Autodesk Inventor part; units mm, degrees
(part 4 of 6)
  line L241 (-272.47, 0.63) -> (-272.9893, 0.63)
  arc A1710 (-273.138, 0.7604) -> (-272.9893, 0.63) centre (-272.9893, 0.78) ccw
  arc A1711 (-273.138, 0.7604) -> (-273.2306, 1.0682) centre (-274.1294, 0.63) ccw
  arc A1712 (-273.2306, 1.0682) -> (-273.7296, 1.38) centre (-273.7294, 0.825) ccw
  arc A1713 (-273.7296, 1.38) -> (-274.2287, 1.0682) centre (-273.7298, 0.825) ccw
  arc A1714 (-274.2287, 1.0682) -> (-274.3213, 0.7604) centre (-273.3298, 0.63) ccw
  arc A1715 (-274.47, 0.63) -> (-274.3213, 0.7604) centre (-274.47, 0.78) ccw
  line L242 (-274.47, 0.63) -> (-274.9893, 0.63)
  arc A1716 (-275.138, 0.7604) -> (-274.9893, 0.63) centre (-274.9893, 0.78) ccw
  arc A1717 (-275.138, 0.7604) -> (-275.2306, 1.0682) centre (-276.1294, 0.63) ccw
  arc A1718 (-275.2306, 1.0682) -> (-275.7296, 1.38) centre (-275.7294, 0.825) ccw
  arc A1719 (-275.7296, 1.38) -> (-276.2287, 1.0682) centre (-275.7298, 0.825) ccw
  arc A1720 (-276.2287, 1.0682) -> (-276.3213, 0.7604) centre (-275.3298, 0.63) ccw
  arc A1721 (-276.47, 0.63) -> (-276.3213, 0.7604) centre (-276.47, 0.78) ccw
  line L243 (-276.47, 0.63) -> (-276.9893, 0.63)
  arc A1722 (-277.138, 0.7604) -> (-276.9893, 0.63) centre (-276.9893, 0.78) ccw
  arc A1723 (-277.138, 0.7604) -> (-277.2306, 1.0682) centre (-278.1294, 0.63) ccw
  arc A1724 (-277.2306, 1.0682) -> (-277.7296, 1.38) centre (-277.7294, 0.825) ccw
  arc A1725 (-277.7296, 1.38) -> (-278.2287, 1.0682) centre (-277.7298, 0.825) ccw
  arc A1726 (-278.2287, 1.0682) -> (-278.3213, 0.7604) centre (-277.3298, 0.63) ccw
  arc A1727 (-278.47, 0.63) -> (-278.3213, 0.7604) centre (-278.47, 0.78) ccw
  line L244 (-278.47, 0.63) -> (-278.9893, 0.63)
  arc A1728 (-279.138, 0.7604) -> (-278.9893, 0.63) centre (-278.9893, 0.78) ccw
  arc A1729 (-279.138, 0.7604) -> (-279.2306, 1.0682) centre (-280.1294, 0.63) ccw
  arc A1730 (-279.2306, 1.0682) -> (-279.7296, 1.38) centre (-279.7294, 0.825) ccw
  arc A1731 (-279.7296, 1.38) -> (-280.2287, 1.0682) centre (-279.7298, 0.825) ccw
  arc A1732 (-280.2287, 1.0682) -> (-280.3213, 0.7604) centre (-279.3298, 0.63) ccw
  arc A1733 (-280.47, 0.63) -> (-280.3213, 0.7604) centre (-280.47, 0.78) ccw
  line L245 (-280.47, 0.63) -> (-280.9893, 0.63)
  arc A1734 (-281.138, 0.7604) -> (-280.9893, 0.63) centre (-280.9893, 0.78) ccw
  arc A1735 (-281.138, 0.7604) -> (-281.2306, 1.0682) centre (-282.1294, 0.63) ccw
  arc A1736 (-281.2306, 1.0682) -> (-281.7296, 1.38) centre (-281.7294, 0.825) ccw
  arc A1737 (-281.7296, 1.38) -> (-282.2287, 1.0682) centre (-281.7298, 0.825) ccw
  arc A1738 (-282.2287, 1.0682) -> (-282.3213, 0.7604) centre (-281.3298, 0.63) ccw
  arc A1739 (-282.47, 0.63) -> (-282.3213, 0.7604) centre (-282.47, 0.78) ccw
  line L246 (-282.47, 0.63) -> (-282.9893, 0.63)
  arc A1740 (-283.138, 0.7604) -> (-282.9893, 0.63) centre (-282.9893, 0.78) ccw
  arc A1741 (-283.138, 0.7604) -> (-283.2306, 1.0682) centre (-284.1294, 0.63) ccw
  arc A1742 (-283.2306, 1.0682) -> (-283.7296, 1.38) centre (-283.7294, 0.825) ccw
  arc A1743 (-283.7296, 1.38) -> (-284.2287, 1.0682) centre (-283.7298, 0.825) ccw
  arc A1744 (-284.2287, 1.0682) -> (-284.3213, 0.7604) centre (-283.3298, 0.63) ccw
  arc A1745 (-284.47, 0.63) -> (-284.3213, 0.7604) centre (-284.47, 0.78) ccw
  line L247 (-284.47, 0.63) -> (-284.9893, 0.63)
  arc A1746 (-285.138, 0.7604) -> (-284.9893, 0.63) centre (-284.9893, 0.78) ccw
  arc A1747 (-285.138, 0.7604) -> (-285.2306, 1.0682) centre (-286.1294, 0.63) ccw
  arc A1748 (-285.2306, 1.0682) -> (-285.7296, 1.38) centre (-285.7294, 0.825) ccw
  arc A1749 (-285.7296, 1.38) -> (-286.2287, 1.0682) centre (-285.7298, 0.825) ccw
  arc A1750 (-286.2287, 1.0682) -> (-286.3213, 0.7604) centre (-285.3298, 0.63) ccw
  arc A1751 (-286.47, 0.63) -> (-286.3213, 0.7604) centre (-286.47, 0.78) ccw
  line L248 (-286.47, 0.63) -> (-286.9893, 0.63)
  arc A1752 (-287.138, 0.7604) -> (-286.9893, 0.63) centre (-286.9893, 0.78) ccw
  arc A1753 (-287.138, 0.7604) -> (-287.2306, 1.0682) centre (-288.1294, 0.63) ccw
  arc A1754 (-287.2306, 1.0682) -> (-287.7296, 1.38) centre (-287.7294, 0.825) ccw
  arc A1755 (-287.7296, 1.38) -> (-288.2287, 1.0682) centre (-287.7298, 0.825) ccw
  arc A1756 (-288.2287, 1.0682) -> (-288.3213, 0.7604) centre (-287.3298, 0.63) ccw
  arc A1757 (-288.47, 0.63) -> (-288.3213, 0.7604) centre (-288.47, 0.78) ccw
  line L249 (-288.47, 0.63) -> (-288.9893, 0.63)
  arc A1758 (-289.138, 0.7604) -> (-288.9893, 0.63) centre (-288.9893, 0.78) ccw
  arc A1759 (-289.138, 0.7604) -> (-289.2306, 1.0682) centre (-290.1294, 0.63) ccw
  arc A1760 (-289.2306, 1.0682) -> (-289.7296, 1.38) centre (-289.7294, 0.825) ccw
  arc A1761 (-289.7296, 1.38) -> (-290.2287, 1.0682) centre (-289.7298, 0.825) ccw
  arc A1762 (-290.2287, 1.0682) -> (-290.3213, 0.7604) centre (-289.3298, 0.63) ccw
  arc A1763 (-290.47, 0.63) -> (-290.3213, 0.7604) centre (-290.47, 0.78) ccw
  line L250 (-290.47, 0.63) -> (-290.9893, 0.63)
  arc A1764 (-291.138, 0.7604) -> (-290.9893, 0.63) centre (-290.9893, 0.78) ccw
  arc A1765 (-291.138, 0.7604) -> (-291.2306, 1.0682) centre (-292.1294, 0.63) ccw
  arc A1766 (-291.2306, 1.0682) -> (-291.7296, 1.38) centre (-291.7294, 0.825) ccw
  arc A1767 (-291.7296, 1.38) -> (-292.2287, 1.0682) centre (-291.7298, 0.825) ccw
  arc A1768 (-292.2287, 1.0682) -> (-292.3213, 0.7604) centre (-291.3298, 0.63) ccw
  arc A1769 (-292.47, 0.63) -> (-292.3213, 0.7604) centre (-292.47, 0.78) ccw
  line L251 (-292.47, 0.63) -> (-292.9893, 0.63)
  arc A1770 (-293.138, 0.7604) -> (-292.9893, 0.63) centre (-292.9893, 0.78) ccw
  arc A1771 (-293.138, 0.7604) -> (-293.2306, 1.0682) centre (-294.1294, 0.63) ccw
  arc A1772 (-293.2306, 1.0682) -> (-293.7296, 1.38) centre (-293.7294, 0.825) ccw
  arc A1773 (-293.7296, 1.38) -> (-294.2287, 1.0682) centre (-293.7298, 0.825) ccw
  arc A1774 (-294.2287, 1.0682) -> (-294.3213, 0.7604) centre (-293.3298, 0.63) ccw
  arc A1775 (-294.47, 0.63) -> (-294.3213, 0.7604) centre (-294.47, 0.78) ccw
  line L252 (-294.47, 0.63) -> (-294.9893, 0.63)
  arc A1776 (-295.138, 0.7604) -> (-294.9893, 0.63) centre (-294.9893, 0.78) ccw
  arc A1777 (-295.138, 0.7604) -> (-295.2306, 1.0682) centre (-296.1294, 0.63) ccw
  arc A1778 (-295.2306, 1.0682) -> (-295.7296, 1.38) centre (-295.7294, 0.825) ccw
  arc A1779 (-295.7296, 1.38) -> (-296.2287, 1.0682) centre (-295.7298, 0.825) ccw
  arc A1780 (-296.2287, 1.0682) -> (-296.3213, 0.7604) centre (-295.3298, 0.63) ccw
  arc A1781 (-296.47, 0.63) -> (-296.3213, 0.7604) centre (-296.47, 0.78) ccw
  line L253 (-296.47, 0.63) -> (-296.9893, 0.63)
  arc A1782 (-297.138, 0.7604) -> (-296.9893, 0.63) centre (-296.9893, 0.78) ccw
  arc A1783 (-297.138, 0.7604) -> (-297.2306, 1.0682) centre (-298.1294, 0.63) ccw
  arc A1784 (-297.2306, 1.0682) -> (-297.7296, 1.38) centre (-297.7294, 0.825) ccw
  arc A1785 (-297.7296, 1.38) -> (-298.2287, 1.0682) centre (-297.7298, 0.825) ccw
  arc A1786 (-298.2287, 1.0682) -> (-298.3213, 0.7604) centre (-297.3298, 0.63) ccw
  arc A1787 (-298.47, 0.63) -> (-298.3213, 0.7604) centre (-298.47, 0.78) ccw
  line L254 (-298.47, 0.63) -> (-298.9893, 0.63)
  arc A1788 (-299.138, 0.7604) -> (-298.9893, 0.63) centre (-298.9893, 0.78) ccw
  arc A1789 (-299.138, 0.7604) -> (-299.2306, 1.0682) centre (-300.1294, 0.63) ccw
  arc A1790 (-299.2306, 1.0682) -> (-299.7296, 1.38) centre (-299.7294, 0.825) ccw
  arc A1791 (-299.7296, 1.38) -> (-300.2287, 1.0682) centre (-299.7298, 0.825) ccw
  arc A1792 (-300.2287, 1.0682) -> (-300.3213, 0.7604) centre (-299.3298, 0.63) ccw
  arc A1793 (-300.47, 0.63) -> (-300.3213, 0.7604) centre (-300.47, 0.78) ccw
  line L255 (-300.47, 0.63) -> (-300.9893, 0.63)
  arc A1794 (-301.138, 0.7604) -> (-300.9893, 0.63) centre (-300.9893, 0.78) ccw
  arc A1795 (-301.138, 0.7604) -> (-301.2306, 1.0682) centre (-302.1294, 0.63) ccw
  arc A1796 (-301.2306, 1.0682) -> (-301.7296, 1.38) centre (-301.7294, 0.825) ccw
  arc A1797 (-301.7296, 1.38) -> (-302.2287, 1.0682) centre (-301.7298, 0.825) ccw
  arc A1798 (-302.2287, 1.0682) -> (-302.3213, 0.7604) centre (-301.3298, 0.63) ccw
  arc A1799 (-302.47, 0.63) -> (-302.3213, 0.7604) centre (-302.47, 0.78) ccw
  line L256 (-302.47, 0.63) -> (-302.9893, 0.63)
  arc A1800 (-303.138, 0.7604) -> (-302.9893, 0.63) centre (-302.9893, 0.78) ccw
  arc A1801 (-303.138, 0.7604) -> (-303.2306, 1.0682) centre (-304.1294, 0.63) ccw
  arc A1802 (-303.2306, 1.0682) -> (-303.7296, 1.38) centre (-303.7294, 0.825) ccw
  arc A1803 (-303.7296, 1.38) -> (-304.2287, 1.0682) centre (-303.7298, 0.825) ccw
  arc A1804 (-304.2287, 1.0682) -> (-304.3213, 0.7604) centre (-303.3298, 0.63) ccw
  arc A1805 (-304.47, 0.63) -> (-304.3213, 0.7604) centre (-304.47, 0.78) ccw
  line L257 (-304.47, 0.63) -> (-304.9893, 0.63)
  arc A1806 (-305.138, 0.7604) -> (-304.9893, 0.63) centre (-304.9893, 0.78) ccw
  arc A1807 (-305.138, 0.7604) -> (-305.2306, 1.0682) centre (-306.1294, 0.63) ccw
  arc A1808 (-305.2306, 1.0682) -> (-305.7296, 1.38) centre (-305.7294, 0.825) ccw
  arc A1809 (-305.7296, 1.38) -> (-306.2287, 1.0682) centre (-305.7298, 0.825) ccw
  arc A1810 (-306.2287, 1.0682) -> (-306.3213, 0.7604) centre (-305.3298, 0.63) ccw
  arc A1811 (-306.47, 0.63) -> (-306.3213, 0.7604) centre (-306.47, 0.78) ccw
  line L258 (-306.47, 0.63) -> (-306.9893, 0.63)
  arc A1812 (-307.138, 0.7604) -> (-306.9893, 0.63) centre (-306.9893, 0.78) ccw
  arc A1813 (-307.138, 0.7604) -> (-307.2306, 1.0682) centre (-308.1294, 0.63) ccw
  arc A1814 (-307.2306, 1.0682) -> (-307.7296, 1.38) centre (-307.7294, 0.825) ccw
  arc A1815 (-307.7296, 1.38) -> (-308.2287, 1.0682) centre (-307.7298, 0.825) ccw
  arc A1816 (-308.2287, 1.0682) -> (-308.3213, 0.7604) centre (-307.3298, 0.63) ccw
  arc A1817 (-308.47, 0.63) -> (-308.3213, 0.7604) centre (-308.47, 0.78) ccw
  line L259 (-308.47, 0.63) -> (-308.9893, 0.63)
  arc A1818 (-309.138, 0.7604) -> (-308.9893, 0.63) centre (-308.9893, 0.78) ccw
  arc A1819 (-309.138, 0.7604) -> (-309.2306, 1.0682) centre (-310.1294, 0.63) ccw
  arc A1820 (-309.2306, 1.0682) -> (-309.7296, 1.38) centre (-309.7294, 0.825) ccw
  arc A1821 (-309.7296, 1.38) -> (-310.2287, 1.0682) centre (-309.7298, 0.825) ccw
  arc A1822 (-310.2287, 1.0682) -> (-310.3213, 0.7604) centre (-309.3298, 0.63) ccw
  arc A1823 (-310.47, 0.63) -> (-310.3213, 0.7604) centre (-310.47, 0.78) ccw
  line L260 (-310.47, 0.63) -> (-310.9893, 0.63)
  arc A1824 (-311.138, 0.7604) -> (-310.9893, 0.63) centre (-310.9893, 0.78) ccw
  arc A1825 (-311.138, 0.7604) -> (-311.2306, 1.0682) centre (-312.1294, 0.63) ccw
  arc A1826 (-311.2306, 1.0682) -> (-311.7296, 1.38) centre (-311.7294, 0.825) ccw
  arc A1827 (-311.7296, 1.38) -> (-312.2287, 1.0682) centre (-311.7298, 0.825) ccw
  arc A1828 (-312.2287, 1.0682) -> (-312.3213, 0.7604) centre (-311.3298, 0.63) ccw
  arc A1829 (-312.47, 0.63) -> (-312.3213, 0.7604) centre (-312.47, 0.78) ccw
  line L261 (-312.47, 0.63) -> (-312.9893, 0.63)
  arc A1830 (-313.138, 0.7604) -> (-312.9893, 0.63) centre (-312.9893, 0.78) ccw
  arc A1831 (-313.138, 0.7604) -> (-313.2306, 1.0682) centre (-314.1294, 0.63) ccw
  arc A1832 (-313.2306, 1.0682) -> (-313.7296, 1.38) centre (-313.7294, 0.825) ccw
  arc A1833 (-313.7296, 1.38) -> (-314.2287, 1.0682) centre (-313.7298, 0.825) ccw
  arc A1834 (-314.2287, 1.0682) -> (-314.3213, 0.7604) centre (-313.3298, 0.63) ccw
  arc A1835 (-314.47, 0.63) -> (-314.3213, 0.7604) centre (-314.47, 0.78) ccw
  line L262 (-314.47, 0.63) -> (-314.9893, 0.63)
  arc A1836 (-315.138, 0.7604) -> (-314.9893, 0.63) centre (-314.9893, 0.78) ccw
  arc A1837 (-315.138, 0.7604) -> (-315.2306, 1.0682) centre (-316.1294, 0.63) ccw
  arc A1838 (-315.2306, 1.0682) -> (-315.7296, 1.38) centre (-315.7294, 0.825) ccw
  arc A1839 (-315.7296, 1.38) -> (-316.2287, 1.0682) centre (-315.7298, 0.825) ccw
  arc A1840 (-316.2287, 1.0682) -> (-316.3213, 0.7604) centre (-315.3298, 0.63) ccw
  arc A1841 (-316.47, 0.63) -> (-316.3213, 0.7604) centre (-316.47, 0.78) ccw
  line L263 (-316.47, 0.63) -> (-316.9893, 0.63)
  arc A1842 (-317.138, 0.7604) -> (-316.9893, 0.63) centre (-316.9893, 0.78) ccw
  arc A1843 (-317.138, 0.7604) -> (-317.2306, 1.0682) centre (-318.1294, 0.63) ccw
  arc A1844 (-317.2306, 1.0682) -> (-317.7296, 1.38) centre (-317.7294, 0.825) ccw
  arc A1845 (-317.7296, 1.38) -> (-318.2287, 1.0682) centre (-317.7298, 0.825) ccw
  arc A1846 (-318.2287, 1.0682) -> (-318.3213, 0.7604) centre (-317.3298, 0.63) ccw
  arc A1847 (-318.47, 0.63) -> (-318.3213, 0.7604) centre (-318.47, 0.78) ccw
  line L264 (-318.47, 0.63) -> (-318.9893, 0.63)
  arc A1848 (-319.138, 0.7604) -> (-318.9893, 0.63) centre (-318.9893, 0.78) ccw
  arc A1849 (-319.138, 0.7604) -> (-319.2306, 1.0682) centre (-320.1294, 0.63) ccw
  arc A1850 (-319.2306, 1.0682) -> (-319.7296, 1.38) centre (-319.7294, 0.825) ccw
  arc A1851 (-319.7296, 1.38) -> (-320.2287, 1.0682) centre (-319.7298, 0.825) ccw
  arc A1852 (-320.2287, 1.0682) -> (-320.3213, 0.7604) centre (-319.3298, 0.63) ccw
  arc A1853 (-320.47, 0.63) -> (-320.3213, 0.7604) centre (-320.47, 0.78) ccw
  line L265 (-320.47, 0.63) -> (-320.9893, 0.63)
  arc A1854 (-321.138, 0.7604) -> (-320.9893, 0.63) centre (-320.9893, 0.78) ccw
  arc A1855 (-321.138, 0.7604) -> (-321.2306, 1.0682) centre (-322.1294, 0.63) ccw
  arc A1856 (-321.2306, 1.0682) -> (-321.7296, 1.38) centre (-321.7294, 0.825) ccw
  arc A1857 (-321.7296, 1.38) -> (-322.2287, 1.0682) centre (-321.7298, 0.825) ccw
  arc A1858 (-322.2287, 1.0682) -> (-322.3213, 0.7604) centre (-321.3298, 0.63) ccw
  arc A1859 (-322.47, 0.63) -> (-322.3213, 0.7604) centre (-322.47, 0.78) ccw
  line L266 (-322.47, 0.63) -> (-322.9893, 0.63)
  arc A1860 (-323.138, 0.7604) -> (-322.9893, 0.63) centre (-322.9893, 0.78) ccw
  arc A1861 (-323.138, 0.7604) -> (-323.2306, 1.0682) centre (-324.1294, 0.63) ccw
  arc A1862 (-323.2306, 1.0682) -> (-323.7296, 1.38) centre (-323.7294, 0.825) ccw
  arc A1863 (-323.7296, 1.38) -> (-324.2287, 1.0682) centre (-323.7298, 0.825) ccw
  arc A1864 (-324.2287, 1.0682) -> (-324.3213, 0.7604) centre (-323.3298, 0.63) ccw
  arc A1865 (-324.47, 0.63) -> (-324.3213, 0.7604) centre (-324.47, 0.78) ccw
  line L267 (-324.47, 0.63) -> (-324.9893, 0.63)
  arc A1866 (-325.138, 0.7604) -> (-324.9893, 0.63) centre (-324.9893, 0.78) ccw
  arc A1867 (-325.138, 0.7604) -> (-325.2306, 1.0682) centre (-326.1294, 0.63) ccw
  arc A1868 (-325.2306, 1.0682) -> (-325.7296, 1.38) centre (-325.7294, 0.825) ccw
  arc A1869 (-325.7296, 1.38) -> (-326.2287, 1.0682) centre (-325.7298, 0.825) ccw
  arc A1870 (-326.2287, 1.0682) -> (-326.3213, 0.7604) centre (-325.3298, 0.63) ccw
  arc A1871 (-326.47, 0.63) -> (-326.3213, 0.7604) centre (-326.47, 0.78) ccw
  line L268 (-326.47, 0.63) -> (-326.9893, 0.63)
  arc A1872 (-327.138, 0.7604) -> (-326.9893, 0.63) centre (-326.9893, 0.78) ccw
  arc A1873 (-327.138, 0.7604) -> (-327.2306, 1.0682) centre (-328.1294, 0.63) ccw
  arc A1874 (-327.2306, 1.0682) -> (-327.7296, 1.38) centre (-327.7294, 0.825) ccw
  arc A1875 (-327.7296, 1.38) -> (-328.2287, 1.0682) centre (-327.7298, 0.825) ccw
  arc A1876 (-328.2287, 1.0682) -> (-328.3213, 0.7604) centre (-327.3298, 0.63) ccw
  arc A1877 (-328.47, 0.63) -> (-328.3213, 0.7604) centre (-328.47, 0.78) ccw
  line L269 (-328.47, 0.63) -> (-328.9893, 0.63)
  arc A1878 (-329.138, 0.7604) -> (-328.9893, 0.63) centre (-328.9893, 0.78) ccw
  arc A1879 (-329.138, 0.7604) -> (-329.2306, 1.0682) centre (-330.1294, 0.63) ccw
  arc A1880 (-329.2306, 1.0682) -> (-329.7296, 1.38) centre (-329.7294, 0.825) ccw
  arc A1881 (-329.7296, 1.38) -> (-330.2287, 1.0682) centre (-329.7298, 0.825) ccw
  arc A1882 (-330.2287, 1.0682) -> (-330.3213, 0.7604) centre (-329.3298, 0.63) ccw
  arc A1883 (-330.47, 0.63) -> (-330.3213, 0.7604) centre (-330.47, 0.78) ccw
  line L270 (-330.47, 0.63) -> (-330.9893, 0.63)
  arc A1884 (-331.138, 0.7604) -> (-330.9893, 0.63) centre (-330.9893, 0.78) ccw
  arc A1885 (-331.138, 0.7604) -> (-331.2306, 1.0682) centre (-332.1294, 0.63) ccw
  arc A1886 (-331.2306, 1.0682) -> (-331.7296, 1.38) centre (-331.7294, 0.825) ccw
  arc A1887 (-331.7296, 1.38) -> (-332.2287, 1.0682) centre (-331.7298, 0.825) ccw
  arc A1888 (-332.2287, 1.0682) -> (-332.3213, 0.7604) centre (-331.3298, 0.63) ccw
  arc A1889 (-332.47, 0.63) -> (-332.3213, 0.7604) centre (-332.47, 0.78) ccw
  line L271 (-332.47, 0.63) -> (-332.9893, 0.63)
  arc A1890 (-333.138, 0.7604) -> (-332.9893, 0.63) centre (-332.9893, 0.78) ccw
  arc A1891 (-333.138, 0.7604) -> (-333.2306, 1.0682) centre (-334.1294, 0.63) ccw
  arc A1892 (-333.2306, 1.0682) -> (-333.7296, 1.38) centre (-333.7294, 0.825) ccw
  arc A1893 (-333.7296, 1.38) -> (-334.2287, 1.0682) centre (-333.7298, 0.825) ccw
  arc A1894 (-334.2287, 1.0682) -> (-334.3213, 0.7604) centre (-333.3298, 0.63) ccw
  arc A1895 (-334.47, 0.63) -> (-334.3213, 0.7604) centre (-334.47, 0.78) ccw
  line L272 (-334.47, 0.63) -> (-334.9893, 0.63)
  arc A1896 (-335.138, 0.7604) -> (-334.9893, 0.63) centre (-334.9893, 0.78) ccw
  arc A1897 (-335.138, 0.7604) -> (-335.2306, 1.0682) centre (-336.1294, 0.63) ccw
  arc A1898 (-335.2306, 1.0682) -> (-335.7296, 1.38) centre (-335.7294, 0.825) ccw
  arc A1899 (-335.7296, 1.38) -> (-336.2287, 1.0682) centre (-335.7298, 0.825) ccw
  arc A1900 (-336.2287, 1.0682) -> (-336.3213, 0.7604) centre (-335.3298, 0.63) ccw
  arc A1901 (-336.47, 0.63) -> (-336.3213, 0.7604) centre (-336.47, 0.78) ccw
  line L273 (-336.47, 0.63) -> (-336.9893, 0.63)
  arc A1902 (-337.138, 0.7604) -> (-336.9893, 0.63) centre (-336.9893, 0.78) ccw
  arc A1903 (-337.138, 0.7604) -> (-337.2306, 1.0682) centre (-338.1294, 0.63) ccw
  arc A1904 (-337.2306, 1.0682) -> (-337.7296, 1.38) centre (-337.7294, 0.825) ccw
  arc A1905 (-337.7296, 1.38) -> (-338.2287, 1.0682) centre (-337.7298, 0.825) ccw
  arc A1906 (-338.2287, 1.0682) -> (-338.3213, 0.7604) centre (-337.3298, 0.63) ccw
  arc A1907 (-338.47, 0.63) -> (-338.3213, 0.7604) centre (-338.47, 0.78) ccw
  line L274 (-338.47, 0.63) -> (-338.9893, 0.63)
  arc A1908 (-339.138, 0.7604) -> (-338.9893, 0.63) centre (-338.9893, 0.78) ccw
  arc A1909 (-339.138, 0.7604) -> (-339.2306, 1.0682) centre (-340.1294, 0.63) ccw
  arc A1910 (-339.2306, 1.0682) -> (-339.7296, 1.38) centre (-339.7294, 0.825) ccw
  arc A1911 (-339.7296, 1.38) -> (-340.2287, 1.0682) centre (-339.7298, 0.825) ccw
  arc A1912 (-340.2287, 1.0682) -> (-340.3213, 0.7604) centre (-339.3298, 0.63) ccw
  arc A1913 (-340.47, 0.63) -> (-340.3213, 0.7604) centre (-340.47, 0.78) ccw
  line L275 (-340.47, 0.63) -> (-340.9893, 0.63)
  arc A1914 (-341.138, 0.7604) -> (-340.9893, 0.63) centre (-340.9893, 0.78) ccw
  arc A1915 (-341.138, 0.7604) -> (-341.2306, 1.0682) centre (-342.1294, 0.63) ccw
  arc A1916 (-341.2306, 1.0682) -> (-341.7296, 1.38) centre (-341.7294, 0.825) ccw
  arc A1917 (-341.7296, 1.38) -> (-342.2287, 1.0682) centre (-341.7298, 0.825) ccw
  arc A1918 (-342.2287, 1.0682) -> (-342.3213, 0.7604) centre (-341.3298, 0.63) ccw
  arc A1919 (-342.47, 0.63) -> (-342.3213, 0.7604) centre (-342.47, 0.78) ccw
  line L276 (-342.47, 0.63) -> (-342.9893, 0.63)
  arc A1920 (-343.138, 0.7604) -> (-342.9893, 0.63) centre (-342.9893, 0.78) ccw
  arc A1921 (-343.138, 0.7604) -> (-343.2306, 1.0682) centre (-344.1294, 0.63) ccw
  arc A1922 (-343.2306, 1.0682) -> (-343.7296, 1.38) centre (-343.7294, 0.825) ccw
  arc A1923 (-343.7296, 1.38) -> (-344.2287, 1.0682) centre (-343.7298, 0.825) ccw
  arc A1924 (-344.2287, 1.0682) -> (-344.3213, 0.7604) centre (-343.3298, 0.63) ccw
  arc A1925 (-344.47, 0.63) -> (-344.3213, 0.7604) centre (-344.47, 0.78) ccw
  line L277 (-344.47, 0.63) -> (-344.9893, 0.63)
  arc A1926 (-345.138, 0.7604) -> (-344.9893, 0.63) centre (-344.9893, 0.78) ccw
  arc A1927 (-345.138, 0.7604) -> (-345.2306, 1.0682) centre (-346.1294, 0.63) ccw
  arc A1928 (-345.2306, 1.0682) -> (-345.7296, 1.38) centre (-345.7294, 0.825) ccw
  arc A1929 (-345.7296, 1.38) -> (-346.2287, 1.0682) centre (-345.7298, 0.825) ccw
  arc A1930 (-346.2287, 1.0682) -> (-346.3213, 0.7604) centre (-345.3298, 0.63) ccw
  arc A1931 (-346.47, 0.63) -> (-346.3213, 0.7604) centre (-346.47, 0.78) ccw
  line L278 (-346.47, 0.63) -> (-346.9893, 0.63)
  arc A1932 (-347.138, 0.7604) -> (-346.9893, 0.63) centre (-346.9893, 0.78) ccw
  arc A1933 (-347.138, 0.7604) -> (-347.2306, 1.0682) centre (-348.1294, 0.63) ccw
  arc A1934 (-347.2306, 1.0682) -> (-347.7296, 1.38) centre (-347.7294, 0.825) ccw
  arc A1935 (-347.7296, 1.38) -> (-348.2287, 1.0682) centre (-347.7298, 0.825) ccw
  arc A1936 (-348.2287, 1.0682) -> (-348.3213, 0.7604) centre (-347.3298, 0.63) ccw
  arc A1937 (-348.47, 0.63) -> (-348.3213, 0.7604) centre (-348.47, 0.78) ccw
  line L279 (-348.47, 0.63) -> (-348.9893, 0.63)
  arc A1938 (-349.138, 0.7604) -> (-348.9893, 0.63) centre (-348.9893, 0.78) ccw
  arc A1939 (-349.138, 0.7604) -> (-349.2306, 1.0682) centre (-350.1294, 0.63) ccw
  arc A1940 (-349.2306, 1.0682) -> (-349.7296, 1.38) centre (-349.7294, 0.825) ccw
  arc A1941 (-349.7296, 1.38) -> (-350.2287, 1.0682) centre (-349.7298, 0.825) ccw
  arc A1942 (-350.2287, 1.0682) -> (-350.3213, 0.7604) centre (-349.3298, 0.63) ccw
  arc A1943 (-350.47, 0.63) -> (-350.3213, 0.7604) centre (-350.47, 0.78) ccw
  line L280 (-350.47, 0.63) -> (-350.9893, 0.63)
  arc A1944 (-351.138, 0.7604) -> (-350.9893, 0.63) centre (-350.9893, 0.78) ccw
  arc A1945 (-351.138, 0.7604) -> (-351.2306, 1.0682) centre (-352.1294, 0.63) ccw
  arc A1946 (-351.2306, 1.0682) -> (-351.7296, 1.38) centre (-351.7294, 0.825) ccw
  arc A1947 (-351.7296, 1.38) -> (-352.2287, 1.0682) centre (-351.7298, 0.825) ccw
  arc A1948 (-352.2287, 1.0682) -> (-352.3213, 0.7604) centre (-351.3298, 0.63) ccw
  arc A1949 (-352.47, 0.63) -> (-352.3213, 0.7604) centre (-352.47, 0.78) ccw
  line L281 (-352.47, 0.63) -> (-352.9893, 0.63)
  arc A1950 (-353.138, 0.7604) -> (-352.9893, 0.63) centre (-352.9893, 0.78) ccw
  arc A1951 (-353.138, 0.7604) -> (-353.2306, 1.0682) centre (-354.1294, 0.63) ccw
  arc A1952 (-353.2306, 1.0682) -> (-353.7296, 1.38) centre (-353.7294, 0.825) ccw
  arc A1953 (-353.7296, 1.38) -> (-354.2287, 1.0682) centre (-353.7298, 0.825) ccw
  arc A1954 (-354.2287, 1.0682) -> (-354.3213, 0.7604) centre (-353.3298, 0.63) ccw
  arc A1955 (-354.47, 0.63) -> (-354.3213, 0.7604) centre (-354.47, 0.78) ccw
  line L282 (-354.47, 0.63) -> (-354.9893, 0.63)
  arc A1956 (-355.138, 0.7604) -> (-354.9893, 0.63) centre (-354.9893, 0.78) ccw
  arc A1957 (-355.138, 0.7604) -> (-355.2306, 1.0682) centre (-356.1294, 0.63) ccw
  arc A1958 (-355.2306, 1.0682) -> (-355.7296, 1.38) centre (-355.7294, 0.825) ccw
  arc A1959 (-355.7296, 1.38) -> (-356.2287, 1.0682) centre (-355.7298, 0.825) ccw
  arc A1960 (-356.2287, 1.0682) -> (-356.3213, 0.7604) centre (-355.3298, 0.63) ccw
  arc A1961 (-356.47, 0.63) -> (-356.3213, 0.7604) centre (-356.47, 0.78) ccw
  line L283 (-356.47, 0.63) -> (-356.9893, 0.63)
  arc A1962 (-357.138, 0.7604) -> (-356.9893, 0.63) centre (-356.9893, 0.78) ccw
  arc A1963 (-357.138, 0.7604) -> (-357.2306, 1.0682) centre (-358.1294, 0.63) ccw
  arc A1964 (-357.2306, 1.0682) -> (-357.7296, 1.38) centre (-357.7294, 0.825) ccw
  arc A1965 (-357.7296, 1.38) -> (-358.2287, 1.0682) centre (-357.7298, 0.825) ccw
  arc A1966 (-358.2287, 1.0682) -> (-358.3213, 0.7604) centre (-357.3298, 0.63) ccw
  arc A1967 (-358.47, 0.63) -> (-358.3213, 0.7604) centre (-358.47, 0.78) ccw
  line L284 (-358.47, 0.63) -> (-358.9893, 0.63)
  arc A1968 (-359.138, 0.7604) -> (-358.9893, 0.63) centre (-358.9893, 0.78) ccw
  arc A1969 (-359.138, 0.7604) -> (-359.2306, 1.0682) centre (-360.1294, 0.63) ccw
  arc A1970 (-359.2306, 1.0682) -> (-359.7296, 1.38) centre (-359.7294, 0.825) ccw
  arc A1971 (-359.7296, 1.38) -> (-360.2287, 1.0682) centre (-359.7298, 0.825) ccw
  arc A1972 (-360.2287, 1.0682) -> (-360.3213, 0.7604) centre (-359.3298, 0.63) ccw
  arc A1973 (-360.47, 0.63) -> (-360.3213, 0.7604) centre (-360.47, 0.78) ccw
  line L285 (-360.47, 0.63) -> (-360.9893, 0.63)
  arc A1974 (-361.138, 0.7604) -> (-360.9893, 0.63) centre (-360.9893, 0.78) ccw
  arc A1975 (-361.138, 0.7604) -> (-361.2306, 1.0682) centre (-362.1294, 0.63) ccw
  arc A1976 (-361.2306, 1.0682) -> (-361.7296, 1.38) centre (-361.7294, 0.825) ccw
  arc A1977 (-361.7296, 1.38) -> (-362.2287, 1.0682) centre (-361.7298, 0.825) ccw
  arc A1978 (-362.2287, 1.0682) -> (-362.3213, 0.7604) centre (-361.3298, 0.63) ccw
  arc A1979 (-362.47, 0.63) -> (-362.3213, 0.7604) centre (-362.47, 0.78) ccw
  line L286 (-362.47, 0.63) -> (-362.9893, 0.63)
  arc A1980 (-363.138, 0.7604) -> (-362.9893, 0.63) centre (-362.9893, 0.78) ccw
  arc A1981 (-363.138, 0.7604) -> (-363.2306, 1.0682) centre (-364.1294, 0.63) ccw
  arc A1982 (-363.2306, 1.0682) -> (-363.7296, 1.38) centre (-363.7294, 0.825) ccw
  arc A1983 (-363.7296, 1.38) -> (-364.2287, 1.0682) centre (-363.7298, 0.825) ccw
  arc A1984 (-364.2287, 1.0682) -> (-364.3213, 0.7604) centre (-363.3298, 0.63) ccw
  arc A1985 (-364.47, 0.63) -> (-364.3213, 0.7604) centre (-364.47, 0.78) ccw
  line L287 (-364.47, 0.63) -> (-364.9893, 0.63)
  arc A1986 (-365.138, 0.7604) -> (-364.9893, 0.63) centre (-364.9893, 0.78) ccw
  arc A1987 (-365.138, 0.7604) -> (-365.2306, 1.0682) centre (-366.1294, 0.63) ccw
  arc A1988 (-365.2306, 1.0682) -> (-365.7296, 1.38) centre (-365.7294, 0.825) ccw
  arc A1989 (-365.7296, 1.38) -> (-366.2287, 1.0682) centre (-365.7298, 0.825) ccw
  arc A1990 (-366.2287, 1.0682) -> (-366.3213, 0.7604) centre (-365.3298, 0.63) ccw
  arc A1991 (-366.47, 0.63) -> (-366.3213, 0.7604) centre (-366.47, 0.78) ccw
  line L288 (-366.47, 0.63) -> (-366.9893, 0.63)
  arc A1992 (-367.138, 0.7604) -> (-366.9893, 0.63) centre (-366.9893, 0.78) ccw
  arc A1993 (-367.138, 0.7604) -> (-367.2306, 1.0682) centre (-368.1294, 0.63) ccw
  arc A1994 (-367.2306, 1.0682) -> (-367.7296, 1.38) centre (-367.7294, 0.825) ccw
  arc A1995 (-367.7296, 1.38) -> (-368.2287, 1.0682) centre (-367.7298, 0.825) ccw
  arc A1996 (-368.2287, 1.0682) -> (-368.3213, 0.7604) centre (-367.3298, 0.63) ccw
  arc A1997 (-368.47, 0.63) -> (-368.3213, 0.7604) centre (-368.47, 0.78) ccw
  line L289 (-368.47, 0.63) -> (-368.9893, 0.63)
  arc A1998 (-369.138, 0.7604) -> (-368.9893, 0.63) centre (-368.9893, 0.78) ccw
  arc A1999 (-369.138, 0.7604) -> (-369.2306, 1.0682) centre (-370.1294, 0.63) ccw
  arc A2000 (-369.2306, 1.0682) -> (-369.7296, 1.38) centre (-369.7294, 0.825) ccw
  arc A2001 (-369.7296, 1.38) -> (-370.2287, 1.0682) centre (-369.7298, 0.825) ccw
  arc A2002 (-370.2287, 1.0682) -> (-370.3213, 0.7604) centre (-369.3298, 0.63) ccw
  arc A2003 (-370.47, 0.63) -> (-370.3213, 0.7604) centre (-370.47, 0.78) ccw
  line L290 (-370.47, 0.63) -> (-370.9893, 0.63)
  arc A2004 (-371.138, 0.7604) -> (-370.9893, 0.63) centre (-370.9893, 0.78) ccw
  arc A2005 (-371.138, 0.7604) -> (-371.2306, 1.0682) centre (-372.1294, 0.63) ccw
  arc A2006 (-371.2306, 1.0682) -> (-371.7296, 1.38) centre (-371.7294, 0.825) ccw
  arc A2007 (-371.7296, 1.38) -> (-372.2287, 1.0682) centre (-371.7298, 0.825) ccw
  arc A2008 (-372.2287, 1.0682) -> (-372.3213, 0.7604) centre (-371.3298, 0.63) ccw
  arc A2009 (-372.47, 0.63) -> (-372.3213, 0.7604) centre (-372.47, 0.78) ccw
  line L291 (-372.47, 0.63) -> (-372.9893, 0.63)
  arc A2010 (-373.138, 0.7604) -> (-372.9893, 0.63) centre (-372.9893, 0.78) ccw
  arc A2011 (-373.138, 0.7604) -> (-373.2306, 1.0682) centre (-374.1294, 0.63) ccw
  arc A2012 (-373.2306, 1.0682) -> (-373.7296, 1.38) centre (-373.7294, 0.825) ccw
  arc A2013 (-373.7296, 1.38) -> (-374.2287, 1.0682) centre (-373.7298, 0.825) ccw
  arc A2014 (-374.2287, 1.0682) -> (-374.3213, 0.7604) centre (-373.3298, 0.63) ccw
  arc A2015 (-374.47, 0.63) -> (-374.3213, 0.7604) centre (-374.47, 0.78) ccw
  line L292 (-374.47, 0.63) -> (-374.9893, 0.63)
  arc A2016 (-375.138, 0.7604) -> (-374.9893, 0.63) centre (-374.9893, 0.78) ccw
  arc A2017 (-375.138, 0.7604) -> (-375.2306, 1.0682) centre (-376.1294, 0.63) ccw
  arc A2018 (-375.2306, 1.0682) -> (-375.7296, 1.38) centre (-375.7294, 0.825) ccw
  arc A2019 (-375.7296, 1.38) -> (-376.2287, 1.0682) centre (-375.7298, 0.825) ccw
  arc A2020 (-376.2287, 1.0682) -> (-376.3213, 0.7604) centre (-375.3298, 0.63) ccw
  arc A2021 (-376.47, 0.63) -> (-376.3213, 0.7604) centre (-376.47, 0.78) ccw
  line L293 (-376.47, 0.63) -> (-376.9893, 0.63)
  arc A2022 (-377.138, 0.7604) -> (-376.9893, 0.63) centre (-376.9893, 0.78) ccw
  arc A2023 (-377.138, 0.7604) -> (-377.2306, 1.0682) centre (-378.1294, 0.63) ccw
  arc A2024 (-377.2306, 1.0682) -> (-377.7296, 1.38) centre (-377.7294, 0.825) ccw
  arc A2025 (-377.7296, 1.38) -> (-378.2287, 1.0682) centre (-377.7298, 0.825) ccw
  arc A2026 (-378.2287, 1.0682) -> (-378.3213, 0.7604) centre (-377.3298, 0.63) ccw
  arc A2027 (-378.47, 0.63) -> (-378.3213, 0.7604) centre (-378.47, 0.78) ccw
  line L294 (-378.47, 0.63) -> (-378.9893, 0.63)
  arc A2028 (-379.138, 0.7604) -> (-378.9893, 0.63) centre (-378.9893, 0.78) ccw
  arc A2029 (-379.138, 0.7604) -> (-379.2306, 1.0682) centre (-380.1294, 0.63) ccw
  arc A2030 (-379.2306, 1.0682) -> (-379.7296, 1.38) centre (-379.7294, 0.825) ccw
  arc A2031 (-379.7296, 1.38) -> (-380.2287, 1.0682) centre (-379.7298, 0.825) ccw
  arc A2032 (-380.2287, 1.0682) -> (-380.3213, 0.7604) centre (-379.3298, 0.63) ccw
  arc A2033 (-380.47, 0.63) -> (-380.3213, 0.7604) centre (-380.47, 0.78) ccw
  line L295 (-380.47, 0.63) -> (-380.9893, 0.63)
  arc A2034 (-381.138, 0.7604) -> (-380.9893, 0.63) centre (-380.9893, 0.78) ccw
  arc A2035 (-381.138, 0.7604) -> (-381.2306, 1.0682) centre (-382.1294, 0.63) ccw
  arc A2036 (-381.2306, 1.0682) -> (-381.7296, 1.38) centre (-381.7294, 0.825) ccw
  arc A2037 (-381.7296, 1.38) -> (-382.2287, 1.0682) centre (-381.7298, 0.825) ccw
  arc A2038 (-382.2287, 1.0682) -> (-382.3213, 0.7604) centre (-381.3298, 0.63) ccw
  arc A2039 (-382.47, 0.63) -> (-382.3213, 0.7604) centre (-382.47, 0.78) ccw
  line L296 (-382.47, 0.63) -> (-382.9893, 0.63)
  arc A2040 (-383.138, 0.7604) -> (-382.9893, 0.63) centre (-382.9893, 0.78) ccw
  arc A2041 (-383.138, 0.7604) -> (-383.2306, 1.0682) centre (-384.1294, 0.63) ccw
  arc A2042 (-383.2306, 1.0682) -> (-383.7296, 1.38) centre (-383.7294, 0.825) ccw
  arc A2043 (-383.7296, 1.38) -> (-384.2287, 1.0682) centre (-383.7298, 0.825) ccw
  arc A2044 (-384.2287, 1.0682) -> (-384.3213, 0.7604) centre (-383.3298, 0.63) ccw
  arc A2045 (-384.47, 0.63) -> (-384.3213, 0.7604) centre (-384.47, 0.78) ccw
  line L297 (-384.47, 0.63) -> (-384.9893, 0.63)
  arc A2046 (-385.138, 0.7604) -> (-384.9893, 0.63) centre (-384.9893, 0.78) ccw
  arc A2047 (-385.138, 0.7604) -> (-385.2306, 1.0682) centre (-386.1294, 0.63) ccw
  arc A2048 (-385.2306, 1.0682) -> (-385.7296, 1.38) centre (-385.7294, 0.825) ccw
  arc A2049 (-385.7296, 1.38) -> (-386.2287, 1.0682) centre (-385.7298, 0.825) ccw
  arc A2050 (-386.2287, 1.0682) -> (-386.3213, 0.7604) centre (-385.3298, 0.63) ccw
  arc A2051 (-386.47, 0.63) -> (-386.3213, 0.7604) centre (-386.47, 0.78) ccw
  line L298 (-386.47, 0.63) -> (-386.9893, 0.63)
  arc A2052 (-387.138, 0.7604) -> (-386.9893, 0.63) centre (-386.9893, 0.78) ccw
  arc A2053 (-387.138, 0.7604) -> (-387.2306, 1.0682) centre (-388.1294, 0.63) ccw
  arc A2054 (-387.2306, 1.0682) -> (-387.7296, 1.38) centre (-387.7294, 0.825) ccw
  arc A2055 (-387.7296, 1.38) -> (-388.2287, 1.0682) centre (-387.7298, 0.825) ccw
  arc A2056 (-388.2287, 1.0682) -> (-388.3213, 0.7604) centre (-387.3298, 0.63) ccw
  arc A2057 (-388.47, 0.63) -> (-388.3213, 0.7604) centre (-388.47, 0.78) ccw
  line L299 (-388.47, 0.63) -> (-388.9893, 0.63)
  arc A2058 (-389.138, 0.7604) -> (-388.9893, 0.63) centre (-388.9893, 0.78) ccw
  arc A2059 (-389.138, 0.7604) -> (-389.2306, 1.0682) centre (-390.1294, 0.63) ccw
  arc A2060 (-389.2306, 1.0682) -> (-389.7296, 1.38) centre (-389.7294, 0.825) ccw
  arc A2061 (-389.7296, 1.38) -> (-390.2287, 1.0682) centre (-389.7298, 0.825) ccw
  arc A2062 (-390.2287, 1.0682) -> (-390.3213, 0.7604) centre (-389.3298, 0.63) ccw
  arc A2063 (-390.47, 0.63) -> (-390.3213, 0.7604) centre (-390.47, 0.78) ccw
  line L300 (-390.47, 0.63) -> (-390.9893, 0.63)
  arc A2064 (-391.138, 0.7604) -> (-390.9893, 0.63) centre (-390.9893, 0.78) ccw
  arc A2065 (-391.138, 0.7604) -> (-391.2306, 1.0682) centre (-392.1294, 0.63) ccw
  arc A2066 (-391.2306, 1.0682) -> (-391.7296, 1.38) centre (-391.7294, 0.825) ccw
  arc A2067 (-391.7296, 1.38) -> (-392.2287, 1.0682) centre (-391.7298, 0.825) ccw
  arc A2068 (-392.2287, 1.0682) -> (-392.3213, 0.7604) centre (-391.3298, 0.63) ccw
  arc A2069 (-392.47, 0.63) -> (-392.3213, 0.7604) centre (-392.47, 0.78) ccw
  line L301 (-392.47, 0.63) -> (-392.9893, 0.63)
  arc A2070 (-393.138, 0.7604) -> (-392.9893, 0.63) centre (-392.9893, 0.78) ccw
  arc A2071 (-393.138, 0.7604) -> (-393.2306, 1.0682) centre (-394.1294, 0.63) ccw
  arc A2072 (-393.2306, 1.0682) -> (-393.7296, 1.38) centre (-393.7294, 0.825) ccw
  arc A2073 (-393.7296, 1.38) -> (-394.2287, 1.0682) centre (-393.7298, 0.825) ccw
  arc A2074 (-394.2287, 1.0682) -> (-394.3213, 0.7604) centre (-393.3298, 0.63) ccw
  arc A2075 (-394.47, 0.63) -> (-394.3213, 0.7604) centre (-394.47, 0.78) ccw
  line L302 (-394.47, 0.63) -> (-394.9893, 0.63)
  arc A2076 (-395.138, 0.7604) -> (-394.9893, 0.63) centre (-394.9893, 0.78) ccw
  arc A2077 (-395.138, 0.7604) -> (-395.2306, 1.0682) centre (-396.1294, 0.63) ccw
  arc A2078 (-395.2306, 1.0682) -> (-395.7296, 1.38) centre (-395.7294, 0.825) ccw
  arc A2079 (-395.7296, 1.38) -> (-396.2287, 1.0682) centre (-395.7298, 0.825) ccw
  arc A2080 (-396.2287, 1.0682) -> (-396.3213, 0.7604) centre (-395.3298, 0.63) ccw
  arc A2081 (-396.47, 0.63) -> (-396.3213, 0.7604) centre (-396.47, 0.78) ccw
  line L303 (-396.47, 0.63) -> (-396.9893, 0.63)
  arc A2082 (-397.138, 0.7604) -> (-396.9893, 0.63) centre (-396.9893, 0.78) ccw
  arc A2083 (-397.138, 0.7604) -> (-397.2306, 1.0682) centre (-398.1294, 0.63) ccw
  arc A2084 (-397.2306, 1.0682) -> (-397.7296, 1.38) centre (-397.7294, 0.825) ccw
  arc A2085 (-397.7296, 1.38) -> (-398.2287, 1.0682) centre (-397.7298, 0.825) ccw
  arc A2086 (-398.2287, 1.0682) -> (-398.3213, 0.7604) centre (-397.3298, 0.63) ccw
  arc A2087 (-398.47, 0.63) -> (-398.3213, 0.7604) centre (-398.47, 0.78) ccw
  line L304 (-398.47, 0.63) -> (-398.9893, 0.63)
  arc A2088 (-399.138, 0.7604) -> (-398.9893, 0.63) centre (-398.9893, 0.78) ccw
  arc A2089 (-399.138, 0.7604) -> (-399.2306, 1.0682) centre (-400.1294, 0.63) ccw
  arc A2090 (-399.2306, 1.0682) -> (-399.7296, 1.38) centre (-399.7294, 0.825) ccw
  arc A2091 (-399.7296, 1.38) -> (-400.2287, 1.0682) centre (-399.7298, 0.825) ccw
  arc A2092 (-400.2287, 1.0682) -> (-400.3213, 0.7604) centre (-399.3298, 0.63) ccw
  arc A2093 (-400.47, 0.63) -> (-400.3213, 0.7604) centre (-400.47, 0.78) ccw
  line L305 (-400.47, 0.63) -> (-400.9893, 0.63)
  arc A2094 (-401.138, 0.7604) -> (-400.9893, 0.63) centre (-400.9893, 0.78) ccw
  arc A2095 (-401.138, 0.7604) -> (-401.2306, 1.0682) centre (-402.1294, 0.63) ccw
  arc A2096 (-401.2306, 1.0682) -> (-401.7296, 1.38) centre (-401.7294, 0.825) ccw
  arc A2097 (-401.7296, 1.38) -> (-402.2287, 1.0682) centre (-401.7298, 0.825) ccw
  arc A2098 (-402.2287, 1.0682) -> (-402.3213, 0.7604) centre (-401.3298, 0.63) ccw
  arc A2099 (-402.47, 0.63) -> (-402.3213, 0.7604) centre (-402.47, 0.78) ccw
  line L306 (-402.47, 0.63) -> (-402.9893, 0.63)
  arc A2100 (-403.138, 0.7604) -> (-402.9893, 0.63) centre (-402.9893, 0.78) ccw
  arc A2101 (-403.138, 0.7604) -> (-403.2306, 1.0682) centre (-404.1294, 0.63) ccw
  arc A2102 (-403.2306, 1.0682) -> (-403.7296, 1.38) centre (-403.7294, 0.825) ccw
  arc A2103 (-403.7296, 1.38) -> (-404.2287, 1.0682) centre (-403.7298, 0.825) ccw
  arc A2104 (-404.2287, 1.0682) -> (-404.3213, 0.7604) centre (-403.3298, 0.63) ccw
  arc A2105 (-404.47, 0.63) -> (-404.3213, 0.7604) centre (-404.47, 0.78) ccw
  line L307 (-404.47, 0.63) -> (-404.9893, 0.63)
  arc A2106 (-405.138, 0.7604) -> (-404.9893, 0.63) centre (-404.9893, 0.78) ccw
  arc A2107 (-405.138, 0.7604) -> (-405.2306, 1.0682) centre (-406.1294, 0.63) ccw
  arc A2108 (-405.2306, 1.0682) -> (-405.7296, 1.38) centre (-405.7294, 0.825) ccw
  arc A2109 (-405.7296, 1.38) -> (-406.2287, 1.0682) centre (-405.7298, 0.825) ccw
  arc A2110 (-406.2287, 1.0682) -> (-406.3213, 0.7604) centre (-405.3298, 0.63) ccw
  arc A2111 (-406.47, 0.63) -> (-406.3213, 0.7604) centre (-406.47, 0.78) ccw
  line L308 (-406.47, 0.63) -> (-406.9893, 0.63)
  arc A2112 (-407.138, 0.7604) -> (-406.9893, 0.63) centre (-406.9893, 0.78) ccw
  arc A2113 (-407.138, 0.7604) -> (-407.2306, 1.0682) centre (-408.1294, 0.63) ccw
  arc A2114 (-407.2306, 1.0682) -> (-407.7296, 1.38) centre (-407.7294, 0.825) ccw
  arc A2115 (-407.7296, 1.38) -> (-408.2287, 1.0682) centre (-407.7298, 0.825) ccw
  arc A2116 (-408.2287, 1.0682) -> (-408.3213, 0.7604) centre (-407.3298, 0.63) ccw
  arc A2117 (-408.47, 0.63) -> (-408.3213, 0.7604) centre (-408.47, 0.78) ccw
  line L309 (-408.47, 0.63) -> (-408.9893, 0.63)
  arc A2118 (-409.138, 0.7604) -> (-408.9893, 0.63) centre (-408.9893, 0.78) ccw
  arc A2119 (-409.138, 0.7604) -> (-409.2306, 1.0682) centre (-410.1294, 0.63) ccw
  arc A2120 (-409.2306, 1.0682) -> (-409.7296, 1.38) centre (-409.7294, 0.825) ccw
  arc A2121 (-409.7296, 1.38) -> (-410.2287, 1.0682) centre (-409.7298, 0.825) ccw
  arc A2122 (-410.2287, 1.0682) -> (-410.3213, 0.7604) centre (-409.3298, 0.63) ccw
  arc A2123 (-410.47, 0.63) -> (-410.3213, 0.7604) centre (-410.47, 0.78) ccw
  line L310 (-410.47, 0.63) -> (-410.9893, 0.63)
  arc A2124 (-411.138, 0.7604) -> (-410.9893, 0.63) centre (-410.9893, 0.78) ccw
  arc A2125 (-411.138, 0.7604) -> (-411.2306, 1.0682) centre (-412.1294, 0.63) ccw
  arc A2126 (-411.2306, 1.0682) -> (-411.7296, 1.38) centre (-411.7294, 0.825) ccw
  arc A2127 (-411.7296, 1.38) -> (-412.2287, 1.0682) centre (-411.7298, 0.825) ccw
  arc A2128 (-412.2287, 1.0682) -> (-412.3213, 0.7604) centre (-411.3298, 0.63) ccw
  arc A2129 (-412.47, 0.63) -> (-412.3213, 0.7604) centre (-412.47, 0.78) ccw
  line L311 (-412.47, 0.63) -> (-412.9893, 0.63)
  arc A2130 (-413.138, 0.7604) -> (-412.9893, 0.63) centre (-412.9893, 0.78) ccw
  arc A2131 (-413.138, 0.7604) -> (-413.2306, 1.0682) centre (-414.1294, 0.63) ccw
  arc A2132 (-413.2306, 1.0682) -> (-413.7296, 1.38) centre (-413.7294, 0.825) ccw
  arc A2133 (-413.7296, 1.38) -> (-414.2287, 1.0682) centre (-413.7298, 0.825) ccw
  arc A2134 (-414.2287, 1.0682) -> (-414.3213, 0.7604) centre (-413.3298, 0.63) ccw
  arc A2135 (-414.47, 0.63) -> (-414.3213, 0.7604) centre (-414.47, 0.78) ccw
  line L312 (-414.47, 0.63) -> (-414.9893, 0.63)
  arc A2136 (-415.138, 0.7604) -> (-414.9893, 0.63) centre (-414.9893, 0.78) ccw
  arc A2137 (-415.138, 0.7604) -> (-415.2306, 1.0682) centre (-416.1294, 0.63) ccw
  arc A2138 (-415.2306, 1.0682) -> (-415.7296, 1.38) centre (-415.7294, 0.825) ccw
  arc A2139 (-415.7296, 1.38) -> (-416.2287, 1.0682) centre (-415.7298, 0.825) ccw
  arc A2140 (-416.2287, 1.0682) -> (-416.3213, 0.7604) centre (-415.3298, 0.63) ccw
  arc A2141 (-416.47, 0.63) -> (-416.3213, 0.7604) centre (-416.47, 0.78) ccw
  line L313 (-416.47, 0.63) -> (-416.9893, 0.63)
  arc A2142 (-417.138, 0.7604) -> (-416.9893, 0.63) centre (-416.9893, 0.78) ccw
  arc A2143 (-417.138, 0.7604) -> (-417.2306, 1.0682) centre (-418.1294, 0.63) ccw
  arc A2144 (-417.2306, 1.0682) -> (-417.7296, 1.38) centre (-417.7294, 0.825) ccw
  arc A2145 (-417.7296, 1.38) -> (-418.2287, 1.0682) centre (-417.7298, 0.825) ccw
  arc A2146 (-418.2287, 1.0682) -> (-418.3213, 0.7604) centre (-417.3298, 0.63) ccw
  arc A2147 (-418.47, 0.63) -> (-418.3213, 0.7604) centre (-418.47, 0.78) ccw
  line L314 (-418.47, 0.63) -> (-418.9893, 0.63)
  arc A2148 (-419.138, 0.7604) -> (-418.9893, 0.63) centre (-418.9893, 0.78) ccw
  arc A2149 (-419.138, 0.7604) -> (-419.2306, 1.0682) centre (-420.1294, 0.63) ccw
  arc A2150 (-419.2306, 1.0682) -> (-419.7296, 1.38) centre (-419.7294, 0.825) ccw
  arc A2151 (-419.7296, 1.38) -> (-420.2287, 1.0682) centre (-419.7298, 0.825) ccw
  arc A2152 (-420.2287, 1.0682) -> (-420.3213, 0.7604) centre (-419.3298, 0.63) ccw
  arc A2153 (-420.47, 0.63) -> (-420.3213, 0.7604) centre (-420.47, 0.78) ccw
  line L315 (-420.47, 0.63) -> (-421.0848, 0.63)
  arc A2154 (-421.1169, 0.7113) -> (-421.0848, 0.63) centre (-420.9674, 0.7233) ccw
  arc A2155 (-421.1169, 0.7113) -> (-421.1937, 1.0234) centre (-422.1137, 0.6314) ccw
  arc A2156 (-421.1937, 1.0234) -> (-421.699, 1.3608) centre (-421.7043, 0.8058) ccw
  arc A2157 (-421.699, 1.3608) -> (-422.1906, 1.074) centre (-421.7047, 0.8058) ccw
  arc A2158 (-422.1906, 1.074) -> (-422.2986, 0.7714) centre (-421.3151, 0.5908) ccw
  arc A2159 (-422.4318, 0.6491) -> (-422.2986, 0.7714) centre (-422.4462, 0.7985) ccw
  arc A2160 (-422.9942, 0.6777) -> (-422.4318, 0.6491) centre (-421.46, 25.315) ccw
  arc A2161 (-423.1143, 0.8128) -> (-422.9942, 0.6777) centre (-422.9648, 0.8248) ccw
  arc A2162 (-423.1143, 0.8128) -> (-423.1912, 1.1249) centre (-424.1111, 0.7329) ccw
  arc A2163 (-423.1912, 1.1249) -> (-423.6511, 1.46) centre (-423.7017, 0.9073) ccw
  arc A2164 (-423.6511, 1.46) -> (-424.188, 1.1756) centre (-423.7021, 0.9074) ccw
  arc A2165 (-424.188, 1.1756) -> (-424.2961, 0.8729) centre (-423.3125, 0.6923) ccw
  arc A2166 (-424.3337, 0.7978) -> (-424.2961, 0.8729) centre (-424.4436, 0.9) ccw
  arc A2167 (-425.0241, 0.8887) -> (-424.3337, 0.7978) centre (-421.46, 25.315) ccw
  arc A2168 (-425.0411, 0.9709) -> (-425.0241, 0.8887) centre (-424.8916, 0.9589) ccw
  arc A2169 (-425.0411, 0.9709) -> (-425.0672, 1.2912) centre (-426.0379, 1.0508) ccw
  arc A2170 (-425.0672, 1.2912) -> (-425.5122, 1.7048) centre (-425.6059, 1.1578) ccw
  arc A2171 (-425.5122, 1.7048) -> (-426.0432, 1.5) centre (-425.6063, 1.1578) ccw
  arc A2172 (-426.0432, 1.5) -> (-426.1982, 1.2185) centre (-425.256, 0.8835) ccw
  arc A2173 (-426.3491, 1.119) -> (-426.1982, 1.2185) centre (-426.3395, 1.2687) ccw
  arc A2174 (-426.8998, 1.2368) -> (-426.3491, 1.119) centre (-421.46, 25.315) ccw
  arc A2175 (-426.9968, 1.3893) -> (-426.8998, 1.2368) centre (-426.8473, 1.3774) ccw
  arc A2176 (-426.9968, 1.3893) -> (-427.023, 1.7097) centre (-427.9936, 1.4692) ccw
  arc A2177 (-427.023, 1.7097) -> (-427.4237, 2.1138) centre (-427.5617, 1.5762) ccw
  arc A2178 (-427.4237, 2.1138) -> (-427.999, 1.9185) centre (-427.562, 1.5763) ccw
  arc A2179 (-427.999, 1.9185) -> (-428.1539, 1.6369) centre (-427.2117, 1.3019) ccw
  arc A2180 (-428.2031, 1.5688) -> (-428.1539, 1.6369) centre (-428.2952, 1.6872) ccw
  arc A2181 (-428.8701, 1.7685) -> (-428.2031, 1.5688) centre (-421.46, 25.315) ccw
  arc A2182 (-428.8738, 1.8524) -> (-428.8701, 1.7685) centre (-428.7281, 1.8167) ccw
  arc A2183 (-428.8738, 1.8524) -> (-428.8486, 2.1728) centre (-429.8452, 2.09) ccw
  arc A2184 (-428.8486, 2.1728) -> (-429.222, 2.652) centre (-429.4017, 2.1269) ccw
  arc A2185 (-429.222, 2.652) -> (-429.7789, 2.5344) centre (-429.402, 2.127) ccw
  arc A2186 (-429.7789, 2.5344) -> (-429.9767, 2.2811) centre (-429.0999, 1.8003) ccw
  arc A2187 (-430.1416, 2.207) -> (-429.9767, 2.2811) centre (-430.1082, 2.3532) ccw
  arc A2188 (-430.6664, 2.411) -> (-430.1416, 2.207) centre (-421.46, 25.315) ccw
  arc A2189 (-430.7379, 2.5771) -> (-430.6664, 2.411) centre (-430.5922, 2.5414) ccw
  arc A2190 (-430.7379, 2.5771) -> (-430.7127, 2.8975) centre (-431.7092, 2.8147) ccw
  arc A2191 (-430.7127, 2.8975) -> (-431.0439, 3.3603) centre (-431.2658, 2.8515) ccw
  arc A2192 (-431.0439, 3.3603) -> (-431.6429, 3.2591) centre (-431.2661, 2.8517) ccw
  arc A2193 (-431.6429, 3.2591) -> (-431.8408, 3.0058) centre (-430.9639, 2.525) ccw
  arc A2194 (-431.9001, 2.9464) -> (-431.8408, 3.0058) centre (-431.9723, 3.0779) ccw
  arc A2195 (-432.5269, 3.2498) -> (-431.9001, 2.9464) centre (-421.46, 25.315) ccw
  arc A2196 (-432.5171, 3.3332) -> (-432.5269, 3.2498) centre (-432.379, 3.2748) ccw
  arc A2197 (-432.5171, 3.3332) -> (-432.4412, 3.6455) centre (-433.4382, 3.7226) ccw
  arc A2198 (-432.4412, 3.6455) -> (-432.7335, 4.1781) centre (-432.9945, 3.6883) ccw
  arc A2199 (-432.7335, 4.1781) -> (-433.302, 4.1507) centre (-432.9949, 3.6885) ccw
  arc A2200 (-433.302, 4.1507) -> (-433.5376, 3.9322) centre (-432.7486, 3.3178) ccw
  arc A2201 (-433.7122, 3.8853) -> (-433.5376, 3.9322) centre (-433.656, 4.0243) ccw
  arc A2202 (-434.1978, 4.1703) -> (-433.7122, 3.8853) centre (-421.46, 25.315) ccw
  arc A2203 (-434.242, 4.3456) -> (-434.1978, 4.1703) centre (-434.1038, 4.2872) ccw
  arc A2204 (-434.242, 4.3456) -> (-434.166, 4.6579) centre (-435.163, 4.735) ccw
  arc A2205 (-434.166, 4.6579) -> (-434.4193, 5.1676) centre (-434.7194, 4.7007) ccw
  arc A2206 (-434.4193, 5.1676) -> (-435.0268, 5.1632) centre (-434.7197, 4.7009) ccw
  arc A2207 (-435.0268, 5.1632) -> (-435.2624, 4.9446) centre (-434.4734, 4.3302) ccw
  arc A2208 (-435.3305, 4.8954) -> (-435.2624, 4.9446) centre (-435.3808, 5.0368) ccw
  arc A2209 (-435.9009, 5.2948) -> (-435.3305, 4.8954) centre (-421.46, 25.315) ccw
  arc A2210 (-435.878, 5.3756) -> (-435.9009, 5.2948) centre (-435.7509, 5.2959) ccw
  arc A2211 (-435.878, 5.3756) -> (-435.7533, 5.6718) centre (-436.7253, 5.9067) ccw
  arc A2212 (-435.7533, 5.6718) -> (-435.957, 6.2441) centre (-436.2927, 5.8022) ccw
  arc A2213 (-435.957, 6.2441) -> (-436.5226, 6.3077) centre (-436.293, 5.8024) ccw
  arc A2214 (-436.5226, 6.3077) -> (-436.79, 6.1295) centre (-436.109, 5.3972) ccw
  arc A2215 (-436.9698, 6.111) -> (-436.79, 6.1295) centre (-436.8922, 6.2393) ccw
  arc A2216 (-437.4038, 6.4698) -> (-436.9698, 6.111) centre (-421.46, 25.315) ccw
  arc A2217 (-437.4195, 6.6499) -> (-437.4038, 6.4698) centre (-437.2924, 6.5702) ccw
  arc A2218 (-437.4195, 6.6499) -> (-437.2948, 6.9461) centre (-438.2668, 7.181) ccw
  arc A2219 (-437.2948, 6.9461) -> (-437.4636, 7.4896) centre (-437.8342, 7.0765) ccw
  arc A2220 (-437.4636, 7.4896) -> (-438.0641, 7.582) centre (-437.8345, 7.0767) ccw
  arc A2221 (-438.0641, 7.582) -> (-438.3315, 7.4038) centre (-437.6505, 6.6715) ccw
  arc A2222 (-438.4066, 7.3661) -> (-438.3315, 7.4038) centre (-438.4337, 7.5136) ccw
  arc A2223 (-438.906, 7.8512) -> (-438.4066, 7.3661) centre (-421.46, 25.315) ccw
  arc A2224 (-438.8706, 7.9273) -> (-438.906, 7.8512) centre (-438.7578, 7.8284) ccw
  arc A2225 (-438.8706, 7.9273) -> (-438.7002, 8.1999) centre (-439.6224, 8.5867) ccw
  arc A2226 (-438.7002, 8.1999) -> (-438.8102, 8.7973) centre (-439.212, 8.4145) ccw
  arc A2227 (-438.8102, 8.7973) -> (-439.3584, 8.9502) centre (-439.2123, 8.4148) ccw
  arc A2228 (-439.3584, 8.9502) -> (-439.6508, 8.8169) centre (-439.0951, 7.9855) ccw
  arc A2229 (-439.8313, 8.8273) -> (-439.6508, 8.8169) centre (-439.7342, 8.9416) ccw
  arc A2230 (-440.2026, 9.2506) -> (-439.8313, 8.8273) centre (-421.46, 25.315) ccw
  arc A2231 (-440.1894, 9.4309) -> (-440.2026, 9.2506) centre (-440.0766, 9.332) ccw
  arc A2232 (-440.1894, 9.4309) -> (-440.019, 9.7034) centre (-440.9412, 10.0903) ccw
  arc A2233 (-440.019, 9.7034) -> (-440.0991, 10.2669) centre (-440.5308, 9.9181) ccw
  arc A2234 (-440.0991, 10.2669) -> (-440.6772, 10.4538) centre (-440.5311, 9.9184) ccw
  arc A2235 (-440.6772, 10.4538) -> (-440.9696, 10.3205) centre (-440.4139, 9.4891) ccw
  arc A2236 (-441.0497, 10.2952) -> (-440.9696, 10.3205) centre (-441.0529, 10.4452) ccw
  arc A2237 (-441.4655, 10.8537) -> (-441.0497, 10.2952) centre (-421.46, 25.315) ccw
  arc A2238 (-441.4184, 10.9232) -> (-441.4655, 10.8537) centre (-441.3228, 10.8076) ccw
  arc A2239 (-441.4184, 10.9232) -> (-441.2068, 11.1651) centre (-442.0555, 11.6939) ccw
  arc A2240 (-441.2068, 11.1651) -> (-441.2201, 11.7725) centre (-441.6778, 11.4586) ccw
  arc A2241 (-441.2201, 11.7725) -> (-441.737, 12.0108) centre (-441.678, 11.4589) ccw
  arc A2242 (-441.737, 12.0108) -> (-442.0469, 11.9257) centre (-441.6308, 11.0164) ccw
  arc A2243 (-442.2234, 11.9648) -> (-442.0469, 11.9257) centre (-442.1093, 12.0621) ccw
  arc A2244 (-442.5225, 12.4418) -> (-442.2234, 11.9648) centre (-421.46, 25.315) ccw
  arc A2245 (-442.4808, 12.6177) -> (-442.5225, 12.4418) centre (-442.3852, 12.5021) ccw
  arc A2246 (-442.4808, 12.6177) -> (-442.2692, 12.8596) centre (-443.1179, 13.3884) ccw
  arc A2247 (-442.2692, 12.8596) -> (-442.2585, 13.4287) centre (-442.7402, 13.1531) ccw
  arc A2248 (-442.2585, 13.4287) -> (-442.7994, 13.7053) centre (-442.7404, 13.1534) ccw
  arc A2249 (-442.7994, 13.7053) -> (-443.1093, 13.6202) centre (-442.6932, 12.7109) ccw
  arc A2250 (-443.1924, 13.6081) -> (-443.1093, 13.6202) centre (-443.1717, 13.7566) ccw
  arc A2251 (-443.5139, 14.2257) -> (-443.1924, 13.6081) centre (-421.46, 25.315) ccw
  arc A2252 (-443.4563, 14.2868) -> (-443.5139, 14.2257) centre (-443.3804, 14.1574) ccw
  arc A2253 (-443.4563, 14.2868) -> (-443.2089, 14.4919) centre (-443.9626, 15.1492) ccw
  arc A2254 (-443.2089, 14.4919) -> (-443.1253, 15.0936) centre (-443.6272, 14.8567) ccw
  arc A2255 (-443.1253, 15.0936) -> (-443.5976, 15.4112) centre (-443.6273, 14.857) ccw
  arc A2256 (-443.5976, 15.4112) -> (-443.9171, 15.3766) centre (-443.6512, 14.4126) ccw
  arc A2257 (-444.0852, 15.4433) -> (-443.9171, 15.3766) centre (-443.957, 15.5212) ccw
  arc A2258 (-444.3044, 15.9619) -> (-444.0852, 15.4433) centre (-421.46, 25.315) ccw
  arc A2259 (-444.2352, 16.1289) -> (-444.3044, 15.9619) centre (-444.1592, 15.9995) ccw
  arc A2260 (-444.2352, 16.1289) -> (-443.9878, 16.334) centre (-444.7414, 16.9913) ccw
  arc A2261 (-443.9878, 16.334) -> (-443.8865, 16.894) centre (-444.406, 16.6988) ccw
  arc A2262 (-443.8865, 16.894) -> (-444.3764, 17.2533) centre (-444.4062, 16.6991) ccw
  arc A2263 (-444.3764, 17.2533) -> (-444.696, 17.2187) centre (-444.43, 16.2548) ccw
  arc A2264 (-444.7799, 17.22) -> (-444.696, 17.2187) centre (-444.7359, 17.3633) ccw
  arc A2265 (-444.999, 17.8809) -> (-444.7799, 17.22) centre (-421.46, 25.315) ccw
  arc A2266 (-444.9324, 17.932) -> (-444.999, 17.8809) centre (-444.878, 17.7922) ccw
  arc A2267 (-444.9324, 17.932) -> (-444.6554, 18.0951) centre (-445.2947, 18.8641) ccw